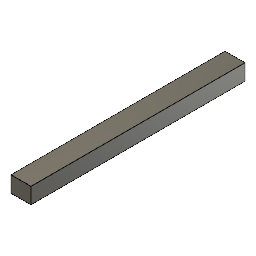
06part (Autodesk Fusion 360 design; units mm, degrees)
Autodesk Fusion 360 part; units mm, degrees
box "BoxPrimitive1" add length 530 width 50 height 40 placed x (0, 0, 1) y (1, 0, 0) z (0, 1, 0) at (0, 0, 0)
